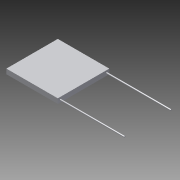
# Autodesk Inventor part: Peltier
Saved by Autodesk Inventor 2014 (Build 180170000, 170)
## iProperties
Created: 2015-04-18
Part Number: Peltier
Material: Generic
Document SubType Name: Modeling
Designer: Owner
Density: 1 g/cm^3
Appearance: White
Author: Owner
Autodesk Inventor part; units mm, degrees
ref_plane "YZ Plane" through (0, 0, 0) normal (1, 0, 0) x (0, 1, 0)
ref_plane "XZ Plane" through (0, 0, 0) normal (0, 1, 0) x (-1, 0, 0)
ref_plane "XY Plane" through (0, 0, 0) normal (0, 0, 1) x (1, 0, 0)
sketch "Sketch1" plane through (0, 0, 0) normal (0, 1, 0) x (-1, 0, 0)
  line L0 (-8.125, 24.375) -> (31.875, 24.375)
  line L1 (31.875, 24.375) -> (31.875, -15.625)
  line L2 (31.875, -15.625) -> (-8.125, -15.625)
  line L3 (-8.125, -15.625) -> (-8.125, 24.375)
  point P0 (0, 0)
  dimension "d0" = 40
  dimension "d1" = 40
  constraints: 8 end point, 2 parallel, 1 horizontal, 1 perpendicular
  measures "d0" distance of L0.end L1.end
  measures "d1" distance of L0.start L0.end
extrude "Extrusion1" add sketch "Sketch1" along normal blind 3.8
sketch "Sketch2" plane through (8.125, 0, 24.375) normal (1, 0, 0) x (0, 0, -1)
  line L0 (40, 0) -> (40, 3.8) projected
  line L1 (0, 0) -> (0, 3.8) projected
  circle A0 centre (2, 1.9) radius 0.5
  circle A1 centre (38, 1.9) radius 0.5
  point P0 (24.375, 0)
  dimension "d4" = 1
  dimension "d5" = 1
  dimension "d6" = 2
  dimension "d7" = 2
  constraints: 2 centre point
  measures "d4" diameter of A0
  measures "d5" diameter of A1
  measures "d6" distance from line of L1 A0.centre
  measures "d7" distance from line of L0 A1.centre
extrude "Extrusion2" add sketch "Sketch2" along normal blind 50
body "Solid1"
